Autodesk Fusion 360 part; units mm, degrees
note: some values were not read from the file. Chosen so that the rebuilt part matches the saved one: which bodies a step acts on.
(part 4 of 4)
  line L205 (7.7875, 59.3875) -> (20.7875, 59.3875)
  arc A172 (21.2875, 58.8875) -> (20.7875, 59.3875) centre (20.7875, 58.8875) ccw
  line L206 (21.2875, 58.8875) -> (21.2875, 45.8875)
  arc A173 (20.7875, 45.3875) -> (21.2875, 45.8875) centre (20.7875, 45.8875) ccw
  line L207 (20.7875, 45.3875) -> (7.7875, 45.3875)
  arc A174 (93.0125, 64.9375) -> (93.5125, 64.4375) centre (93.5125, 64.9375) ccw
  line L208 (93.0125, 64.9375) -> (93.0125, 77.9375)
  arc A175 (93.5125, 78.4375) -> (93.0125, 77.9375) centre (93.5125, 77.9375) ccw
  line L209 (93.5125, 78.4375) -> (106.5125, 78.4375)
  arc A176 (107.0125, 77.9375) -> (106.5125, 78.4375) centre (106.5125, 77.9375) ccw
  line L210 (107.0125, 77.9375) -> (107.0125, 64.9375)
  arc A177 (106.5125, 64.4375) -> (107.0125, 64.9375) centre (106.5125, 64.9375) ccw
  line L211 (106.5125, 64.4375) -> (93.5125, 64.4375)
  arc A178 (35.8625, 64.9375) -> (36.3625, 64.4375) centre (36.3625, 64.9375) ccw
  line L212 (35.8625, 64.9375) -> (35.8625, 77.9375)
  arc A179 (36.3625, 78.4375) -> (35.8625, 77.9375) centre (36.3625, 77.9375) ccw
  line L213 (36.3625, 78.4375) -> (49.3625, 78.4375)
  arc A180 (49.8625, 77.9375) -> (49.3625, 78.4375) centre (49.3625, 77.9375) ccw
  line L214 (49.8625, 77.9375) -> (49.8625, 64.9375)
  arc A181 (49.3625, 64.4375) -> (49.8625, 64.9375) centre (49.3625, 64.9375) ccw
  line L215 (49.3625, 64.4375) -> (36.3625, 64.4375)
  arc A182 (131.1125, 64.9375) -> (131.6125, 64.4375) centre (131.6125, 64.9375) ccw
  line L216 (131.1125, 64.9375) -> (131.1125, 77.9375)
  arc A183 (131.6125, 78.4375) -> (131.1125, 77.9375) centre (131.6125, 77.9375) ccw
  line L217 (131.6125, 78.4375) -> (144.6125, 78.4375)
  arc A184 (145.1125, 77.9375) -> (144.6125, 78.4375) centre (144.6125, 77.9375) ccw
  line L218 (145.1125, 77.9375) -> (145.1125, 64.9375)
  arc A185 (144.6125, 64.4375) -> (145.1125, 64.9375) centre (144.6125, 64.9375) ccw
  line L219 (144.6125, 64.4375) -> (131.6125, 64.4375)
  arc A186 (28.7187, 103.0375) -> (29.2188, 102.5375) centre (29.2188, 103.0375) ccw
  line L220 (28.7187, 103.0375) -> (28.7188, 116.0375)
  arc A187 (29.2188, 116.5375) -> (28.7188, 116.0375) centre (29.2188, 116.0375) ccw
  line L221 (29.2188, 116.5375) -> (42.2188, 116.5375)
  arc A188 (42.7188, 116.0375) -> (42.2188, 116.5375) centre (42.2188, 116.0375) ccw
  line L222 (42.7188, 116.0375) -> (42.7188, 103.0375)
  arc A189 (42.2188, 102.5375) -> (42.7188, 103.0375) centre (42.2188, 103.0375) ccw
  line L223 (42.2188, 102.5375) -> (29.2188, 102.5375)
  arc A190 (31.1, 45.8875) -> (31.6, 45.3875) centre (31.6, 45.8875) ccw
  line L224 (31.1, 45.8875) -> (31.1, 58.8875)
  arc A191 (31.6, 59.3875) -> (31.1, 58.8875) centre (31.6, 58.8875) ccw
  line L225 (31.6, 59.3875) -> (44.6, 59.3875)
  arc A192 (45.1, 58.8875) -> (44.6, 59.3875) centre (44.6, 58.8875) ccw
  line L226 (45.1, 58.8875) -> (45.1, 45.8875)
  arc A193 (44.6, 45.3875) -> (45.1, 45.8875) centre (44.6, 45.8875) ccw
  line L227 (44.6, 45.3875) -> (31.6, 45.3875)
  arc A194 (59.675, 26.8375) -> (60.175, 26.3375) centre (60.175, 26.8375) ccw
  line L228 (59.675, 26.8375) -> (59.675, 39.8375)
  arc A195 (60.175, 40.3375) -> (59.675, 39.8375) centre (60.175, 39.8375) ccw
  line L229 (60.175, 40.3375) -> (73.175, 40.3375)
  arc A196 (73.675, 39.8375) -> (73.175, 40.3375) centre (73.175, 39.8375) ccw
  line L230 (73.675, 39.8375) -> (73.675, 26.8375)
  arc A197 (73.175, 26.3375) -> (73.675, 26.8375) centre (73.175, 26.8375) ccw
  line L231 (73.175, 26.3375) -> (60.175, 26.3375)
  arc A198 (2.525, 26.8375) -> (3.025, 26.3375) centre (3.025, 26.8375) ccw
  line L232 (2.525, 26.8375) -> (2.525, 39.8375)
  arc A199 (3.025, 40.3375) -> (2.525, 39.8375) centre (3.025, 39.8375) ccw
  line L233 (3.025, 40.3375) -> (16.025, 40.3375)
  arc A200 (16.525, 39.8375) -> (16.025, 40.3375) centre (16.025, 39.8375) ccw
  line L234 (16.525, 39.8375) -> (16.525, 26.8375)
  arc A201 (16.025, 26.3375) -> (16.525, 26.8375) centre (16.025, 26.8375) ccw
  line L235 (16.025, 26.3375) -> (3.025, 26.3375)
  line L236 (2.3022, 101.2599) -> (40.5603, 101.2599)
  line L237 (40.5603, 101.2599) -> (40.5603, 80.4875)
  line L238 (40.5603, 80.4875) -> (2.3022, 80.4875)
  line L239 (2.3022, 80.4875) -> (2.3022, 101.2599)
  line L240 (79.4039, 119.5375) -> (192.9223, 119.5375)
  line L241 (192.9223, 119.5375) -> (192.9223, 99.5375)
  line L242 (192.9223, 99.5375) -> (79.4039, 99.5375)
  line L243 (79.4039, 99.5375) -> (79.4039, 119.5375)
  line L244 (189.9223, 107.7515) -> (189.9223, 110.0455)
  line L245 (245.1898, 82.2099) -> (283.4478, 82.2099)
  line L246 (283.4478, 82.2099) -> (283.4478, 61.4375)
  line L247 (283.4478, 61.4375) -> (245.1898, 61.4375)
  line L248 (245.1898, 61.4375) -> (245.1898, 82.2099)
  line L249 (248.1898, 71.9455) -> (248.1898, 69.6515)
  line L250 (253.4048, 79.2099) -> (251.3568, 79.2099)
  line L251 (280.4478, 69.6515) -> (280.4478, 71.9455)
  line L252 (257.8188, 64.4375) -> (270.8188, 64.4375)
  line L253 (247.571, 42.896) -> (285.829, 42.896)
  line L254 (285.829, 42.896) -> (285.829, 23.3375)
  line L255 (285.829, 23.3375) -> (247.571, 23.3375)
  line L256 (247.571, 23.3375) -> (247.571, 42.896)
  line L257 (250.571, 33.8455) -> (250.571, 31.5515)
  line L258 (282.829, 31.5515) -> (282.829, 33.8455)
  line L259 (279.662, 41.1099) -> (277.614, 41.1099)
  line L260 (260.2, 26.3375) -> (273.2, 26.3375)
  dimension "d40" = 3
  dimension "d41" = 3
  dimension "d43" = 3
  dimension "d44" = 3
  dimension "d45" = 3
  dimension "d46" = 3
  dimension "d47" = 3
  dimension "d48" = 3
  dimension "d50" = 3
  dimension "d51" = 3
  dimension "d52" = 3
  dimension "d53" = 3
  dimension "d54" = 3
  dimension "d55" = 3
  dimension "d56" = 1.7861
  dimension "d57" = 3
  constraint horizontal L236
  constraint vertical L237
  constraint horizontal L238
  constraint vertical L239
  constraint horizontal L240
  constraint vertical L241
  constraint horizontal L242
  constraint vertical L243
  constraint horizontal L245
  constraint vertical L246
  constraint horizontal L247
  constraint vertical L248
  constraint horizontal L253
  constraint vertical L254
  constraint horizontal L255
  constraint vertical L256
  measures "d40" distance of L108 L238
  measures "d41" distance of L115 L239
  measures "d43" distance of L120 L236
  measures "d44" distance of L101 L237
  measures "d45" distance of L3 L242
  measures "d46" distance of L12 L243
  measures "d47" distance of L21 L240
  measures "d48" distance of L241 L244
  measures "d50" distance of L248 L249
  measures "d51" distance of L245 L250
  measures "d52" distance of L246 L251
  measures "d53" distance of L247 L252
  measures "d54" distance of L256 L257
  measures "d55" distance of L254 L258
  measures "d56" distance of L253 L259
  measures "d57" distance of L255 L260
extrude "Extrude2" cut sketch "Sketch3" against normal blind 1.5 contours L0 L1 L2 A0 L3 A1 L4 L5 A2 L6 A3 L7 A4 L8 L9 A5 L10 L11 A6 L12 A7 L13 A8 L14 A9 L15 A10 L16 A11 L17 A12 L18 A13 L19 L20 A14 L21 A15 L22 L23 L24 L240 L242 L243 | L0 L1 L2 A0 L3 A1 L4 L5 A2 L6 A3 L7 A4 L8 L9 A5 L10 L11 A6 L12 A7 L13 A8 L14 A9 L15 A10 L16 A11 L17 A12 L18 A13 L19 L20 A14 L21 A15 L22 L23 L24 L240 L241 L242 | L236 L237 L238 L239 | L245 L246 L247 L248 | L253 L254 L255 L256 bodies 1 2
sketch "Sketch4" plane through (0, 0, 0) normal (0, 0, -1) x (1, 0, 0)
  arc A0 (2.525, 26.8375) -> (3.025, 26.3375) centre (3.025, 26.8375) ccw
  line L0 (2.525, 26.8375) -> (2.525, 39.8375)
  arc A1 (3.025, 40.3375) -> (2.525, 39.8375) centre (3.025, 39.8375) ccw
  line L1 (3.025, 40.3375) -> (16.025, 40.3375)
  arc A2 (16.525, 39.8375) -> (16.025, 40.3375) centre (16.025, 39.8375) ccw
  line L2 (16.525, 39.8375) -> (16.525, 26.8375)
  arc A3 (16.025, 26.3375) -> (16.525, 26.8375) centre (16.025, 26.8375) ccw
  line L3 (16.025, 26.3375) -> (3.025, 26.3375)
  arc A4 (59.675, 26.8375) -> (60.175, 26.3375) centre (60.175, 26.8375) ccw
  line L4 (59.675, 26.8375) -> (59.675, 39.8375)
  arc A5 (60.175, 40.3375) -> (59.675, 39.8375) centre (60.175, 39.8375) ccw
  line L5 (60.175, 40.3375) -> (73.175, 40.3375)
  arc A6 (73.675, 39.8375) -> (73.175, 40.3375) centre (73.175, 39.8375) ccw
  line L6 (73.675, 39.8375) -> (73.675, 26.8375)
  arc A7 (73.175, 26.3375) -> (73.675, 26.8375) centre (73.175, 26.8375) ccw
  line L7 (73.175, 26.3375) -> (60.175, 26.3375)
  arc A8 (31.1, 45.8875) -> (31.6, 45.3875) centre (31.6, 45.8875) ccw
  line L8 (31.1, 45.8875) -> (31.1, 58.8875)
  arc A9 (31.6, 59.3875) -> (31.1, 58.8875) centre (31.6, 58.8875) ccw
  line L9 (31.6, 59.3875) -> (44.6, 59.3875)
  arc A10 (45.1, 58.8875) -> (44.6, 59.3875) centre (44.6, 58.8875) ccw
  line L10 (45.1, 58.8875) -> (45.1, 45.8875)
  arc A11 (44.6, 45.3875) -> (45.1, 45.8875) centre (44.6, 45.8875) ccw
  line L11 (44.6, 45.3875) -> (31.6, 45.3875)
  arc A12 (28.7187, 103.0375) -> (29.2188, 102.5375) centre (29.2188, 103.0375) ccw
  line L12 (28.7187, 103.0375) -> (28.7188, 116.0375)
  arc A13 (29.2188, 116.5375) -> (28.7188, 116.0375) centre (29.2188, 116.0375) ccw
  line L13 (29.2188, 116.5375) -> (42.2188, 116.5375)
  arc A14 (42.7188, 116.0375) -> (42.2188, 116.5375) centre (42.2188, 116.0375) ccw
  line L14 (42.7188, 116.0375) -> (42.7188, 103.0375)
  arc A15 (42.2188, 102.5375) -> (42.7188, 103.0375) centre (42.2188, 103.0375) ccw
  line L15 (42.2188, 102.5375) -> (29.2188, 102.5375)
  arc A16 (131.1125, 64.9375) -> (131.6125, 64.4375) centre (131.6125, 64.9375) ccw
  line L16 (131.1125, 64.9375) -> (131.1125, 77.9375)
  arc A17 (131.6125, 78.4375) -> (131.1125, 77.9375) centre (131.6125, 77.9375) ccw
  line L17 (131.6125, 78.4375) -> (144.6125, 78.4375)
  arc A18 (145.1125, 77.9375) -> (144.6125, 78.4375) centre (144.6125, 77.9375) ccw
  line L18 (145.1125, 77.9375) -> (145.1125, 64.9375)
  arc A19 (144.6125, 64.4375) -> (145.1125, 64.9375) centre (144.6125, 64.9375) ccw
  line L19 (144.6125, 64.4375) -> (131.6125, 64.4375)
  arc A20 (35.8625, 64.9375) -> (36.3625, 64.4375) centre (36.3625, 64.9375) ccw
  line L20 (35.8625, 64.9375) -> (35.8625, 77.9375)
  arc A21 (36.3625, 78.4375) -> (35.8625, 77.9375) centre (36.3625, 77.9375) ccw
  line L21 (36.3625, 78.4375) -> (49.3625, 78.4375)
  arc A22 (49.8625, 77.9375) -> (49.3625, 78.4375) centre (49.3625, 77.9375) ccw
  line L22 (49.8625, 77.9375) -> (49.8625, 64.9375)
  arc A23 (49.3625, 64.4375) -> (49.8625, 64.9375) centre (49.3625, 64.9375) ccw
  line L23 (49.3625, 64.4375) -> (36.3625, 64.4375)
  arc A24 (93.0125, 64.9375) -> (93.5125, 64.4375) centre (93.5125, 64.9375) ccw
  line L24 (93.0125, 64.9375) -> (93.0125, 77.9375)
  arc A25 (93.5125, 78.4375) -> (93.0125, 77.9375) centre (93.5125, 77.9375) ccw
  line L25 (93.5125, 78.4375) -> (106.5125, 78.4375)
  arc A26 (107.0125, 77.9375) -> (106.5125, 78.4375) centre (106.5125, 77.9375) ccw
  line L26 (107.0125, 77.9375) -> (107.0125, 64.9375)
  arc A27 (106.5125, 64.4375) -> (107.0125, 64.9375) centre (106.5125, 64.9375) ccw
  line L27 (106.5125, 64.4375) -> (93.5125, 64.4375)
  arc A28 (7.2875, 45.8875) -> (7.7875, 45.3875) centre (7.7875, 45.8875) ccw
  line L28 (7.2875, 45.8875) -> (7.2875, 58.8875)
  arc A29 (7.7875, 59.3875) -> (7.2875, 58.8875) centre (7.7875, 58.8875) ccw
  line L29 (7.7875, 59.3875) -> (20.7875, 59.3875)
  arc A30 (21.2875, 58.8875) -> (20.7875, 59.3875) centre (20.7875, 58.8875) ccw
  line L30 (21.2875, 58.8875) -> (21.2875, 45.8875)
  arc A31 (20.7875, 45.3875) -> (21.2875, 45.8875) centre (20.7875, 45.8875) ccw
  line L31 (20.7875, 45.3875) -> (7.7875, 45.3875)
  arc A32 (135.875, 26.8375) -> (136.375, 26.3375) centre (136.375, 26.8375) ccw
  line L32 (135.875, 26.8375) -> (135.875, 39.8375)
  arc A33 (136.375, 40.3375) -> (135.875, 39.8375) centre (136.375, 39.8375) ccw
  line L33 (136.375, 40.3375) -> (149.375, 40.3375)
  arc A34 (149.875, 39.8375) -> (149.375, 40.3375) centre (149.375, 39.8375) ccw
  line L34 (149.875, 39.8375) -> (149.875, 26.8375)
  arc A35 (149.375, 26.3375) -> (149.875, 26.8375) centre (149.375, 26.8375) ccw
  line L35 (149.375, 26.3375) -> (136.375, 26.3375)
  arc A36 (35.8625, 3.025) -> (36.3625, 2.525) centre (36.3625, 3.025) ccw
  line L36 (35.8625, 3.025) -> (35.8625, 16.025)
  arc A37 (36.3625, 16.525) -> (35.8625, 16.025) centre (36.3625, 16.025) ccw
  line L37 (36.3625, 16.525) -> (49.3625, 16.525)
  arc A38 (49.8625, 16.025) -> (49.3625, 16.525) centre (49.3625, 16.025) ccw
  line L38 (49.8625, 16.025) -> (49.8625, 3.025)
  arc A39 (49.3625, 2.525) -> (49.8625, 3.025) centre (49.3625, 3.025) ccw
  line L39 (49.3625, 2.525) -> (36.3625, 2.525)
  arc A40 (73.9625, 64.9375) -> (74.4625, 64.4375) centre (74.4625, 64.9375) ccw
  line L40 (73.9625, 64.9375) -> (73.9625, 77.9375)
  arc A41 (74.4625, 78.4375) -> (73.9625, 77.9375) centre (74.4625, 77.9375) ccw
  line L41 (74.4625, 78.4375) -> (87.4625, 78.4375)
  arc A42 (87.9625, 77.9375) -> (87.4625, 78.4375) centre (87.4625, 77.9375) ccw
  line L42 (87.9625, 77.9375) -> (87.9625, 64.9375)
  arc A43 (87.4625, 64.4375) -> (87.9625, 64.9375) centre (87.4625, 64.9375) ccw
  line L43 (87.4625, 64.4375) -> (74.4625, 64.4375)
  arc A44 (54.9125, 64.9375) -> (55.4125, 64.4375) centre (55.4125, 64.9375) ccw
  line L44 (54.9125, 64.9375) -> (54.9125, 77.9375)
  arc A45 (55.4125, 78.4375) -> (54.9125, 77.9375) centre (55.4125, 77.9375) ccw
  line L45 (55.4125, 78.4375) -> (68.4125, 78.4375)
  arc A46 (68.9125, 77.9375) -> (68.4125, 78.4375) centre (68.4125, 77.9375) ccw
  line L46 (68.9125, 77.9375) -> (68.9125, 64.9375)
  arc A47 (68.4125, 64.4375) -> (68.9125, 64.9375) centre (68.4125, 64.9375) ccw
  line L47 (68.4125, 64.4375) -> (55.4125, 64.4375)
  arc A48 (126.35, 45.8875) -> (126.85, 45.3875) centre (126.85, 45.8875) ccw
  line L48 (126.35, 45.8875) -> (126.35, 58.8875)
  arc A49 (126.85, 59.3875) -> (126.35, 58.8875) centre (126.85, 58.8875) ccw
  line L49 (126.85, 59.3875) -> (139.85, 59.3875)
  arc A50 (140.35, 58.8875) -> (139.85, 59.3875) centre (139.85, 58.8875) ccw
  line L50 (140.35, 58.8875) -> (140.35, 45.8875)
  arc A51 (139.85, 45.3875) -> (140.35, 45.8875) centre (139.85, 45.8875) ccw
  line L51 (139.85, 45.3875) -> (126.85, 45.3875)
  arc A52 (116.825, 26.8375) -> (117.325, 26.3375) centre (117.325, 26.8375) ccw
  line L52 (116.825, 26.8375) -> (116.825, 39.8375)
  arc A53 (117.325, 40.3375) -> (116.825, 39.8375) centre (117.325, 39.8375) ccw
  line L53 (117.325, 40.3375) -> (130.325, 40.3375)
  arc A54 (130.825, 39.8375) -> (130.325, 40.3375) centre (130.325, 39.8375) ccw
  line L54 (130.825, 39.8375) -> (130.825, 26.8375)
  arc A55 (130.325, 26.3375) -> (130.825, 26.8375) centre (130.325, 26.8375) ccw
  line L55 (130.325, 26.3375) -> (117.325, 26.3375)
  arc A56 (107.3, 45.8875) -> (107.8, 45.3875) centre (107.8, 45.8875) ccw
  line L56 (107.3, 45.8875) -> (107.3, 58.8875)
  arc A57 (107.8, 59.3875) -> (107.3, 58.8875) centre (107.8, 58.8875) ccw
  line L57 (107.8, 59.3875) -> (120.8, 59.3875)
  arc A58 (121.3, 58.8875) -> (120.8, 59.3875) centre (120.8, 58.8875) ccw
  line L58 (121.3, 58.8875) -> (121.3, 45.8875)
  arc A59 (120.8, 45.3875) -> (121.3, 45.8875) centre (120.8, 45.8875) ccw
  line L59 (120.8, 45.3875) -> (107.8, 45.3875)
  arc A60 (54.9125, 3.025) -> (55.4125, 2.525) centre (55.4125, 3.025) ccw
  line L60 (54.9125, 3.025) -> (54.9125, 16.025)
  arc A61 (55.4125, 16.525) -> (54.9125, 16.025) centre (55.4125, 16.025) ccw
  line L61 (55.4125, 16.525) -> (68.4125, 16.525)
  arc A62 (68.9125, 16.025) -> (68.4125, 16.525) centre (68.4125, 16.025) ccw
  line L62 (68.9125, 16.025) -> (68.9125, 3.025)
  arc A63 (68.4125, 2.525) -> (68.9125, 3.025) centre (68.4125, 3.025) ccw
  line L63 (68.4125, 2.525) -> (55.4125, 2.525)
  arc A64 (145.4, 45.8875) -> (145.9, 45.3875) centre (145.9, 45.8875) ccw
  line L64 (145.4, 45.8875) -> (145.4, 58.8875)
  arc A65 (145.9, 59.3875) -> (145.4, 58.8875) centre (145.9, 58.8875) ccw
  line L65 (145.9, 59.3875) -> (158.9, 59.3875)
  arc A66 (159.4, 58.8875) -> (158.9, 59.3875) centre (158.9, 58.8875) ccw
  line L66 (159.4, 58.8875) -> (159.4, 45.8875)
  arc A67 (158.9, 45.3875) -> (159.4, 45.8875) centre (158.9, 45.8875) ccw
  line L67 (158.9, 45.3875) -> (145.9, 45.3875)
  arc A68 (93.0125, 3.025) -> (93.5125, 2.525) centre (93.5125, 3.025) ccw
  line L68 (93.0125, 3.025) -> (93.0125, 16.025)
  arc A69 (93.5125, 16.525) -> (93.0125, 16.025) centre (93.5125, 16.025) ccw
  line L69 (93.5125, 16.525) -> (106.5125, 16.525)
  arc A70 (107.0125, 16.025) -> (106.5125, 16.525) centre (106.5125, 16.025) ccw
  line L70 (107.0125, 16.025) -> (107.0125, 3.025)
  arc A71 (106.5125, 2.525) -> (107.0125, 3.025) centre (106.5125, 3.025) ccw
  line L71 (106.5125, 2.525) -> (93.5125, 2.525)
  arc A72 (73.9625, 3.025) -> (74.4625, 2.525) centre (74.4625, 3.025) ccw
  line L72 (73.9625, 3.025) -> (73.9625, 16.025)
  arc A73 (74.4625, 16.525) -> (73.9625, 16.025) centre (74.4625, 16.025) ccw
  line L73 (74.4625, 16.525) -> (87.4625, 16.525)
  arc A74 (87.9625, 16.025) -> (87.4625, 16.525) centre (87.4625, 16.025) ccw
  line L74 (87.9625, 16.025) -> (87.9625, 3.025)
  arc A75 (87.4625, 2.525) -> (87.9625, 3.025) centre (87.4625, 3.025) ccw
  line L75 (87.4625, 2.525) -> (74.4625, 2.525)
  arc A76 (2.525, 3.025) -> (3.025, 2.525) centre (3.025, 3.025) ccw
  line L76 (2.525, 3.025) -> (2.525, 16.025)
  arc A77 (3.025, 16.525) -> (2.525, 16.025) centre (3.025, 16.025) ccw
  line L77 (3.025, 16.525) -> (16.025, 16.525)
  arc A78 (16.525, 16.025) -> (16.025, 16.525) centre (16.025, 16.025) ccw
  line L78 (16.525, 16.025) -> (16.525, 3.025)
  arc A79 (16.025, 2.525) -> (16.525, 3.025) centre (16.025, 3.025) ccw
  line L79 (16.025, 2.525) -> (3.025, 2.525)
  arc A80 (140.6375, 3.025) -> (141.1375, 2.525) centre (141.1375, 3.025) ccw
  line L80 (140.6375, 3.025) -> (140.6375, 16.025)
  arc A81 (141.1375, 16.525) -> (140.6375, 16.025) centre (141.1375, 16.025) ccw
  line L81 (141.1375, 16.525) -> (154.1375, 16.525)
  arc A82 (154.6375, 16.025) -> (154.1375, 16.525) centre (154.1375, 16.025) ccw
  line L82 (154.6375, 16.025) -> (154.6375, 3.025)
  arc A83 (154.1375, 2.525) -> (154.6375, 3.025) centre (154.1375, 3.025) ccw
  line L83 (154.1375, 2.525) -> (141.1375, 2.525)
  arc A84 (78.725, 26.8375) -> (79.225, 26.3375) centre (79.225, 26.8375) ccw
  line L84 (78.725, 26.8375) -> (78.725, 39.8375)
  arc A85 (79.225, 40.3375) -> (78.725, 39.8375) centre (79.225, 39.8375) ccw
  line L85 (79.225, 40.3375) -> (92.225, 40.3375)
  arc A86 (92.725, 39.8375) -> (92.225, 40.3375) centre (92.225, 39.8375) ccw
  line L86 (92.725, 39.8375) -> (92.725, 26.8375)
  arc A87 (92.225, 26.3375) -> (92.725, 26.8375) centre (92.225, 26.8375) ccw
  line L87 (92.225, 26.3375) -> (79.225, 26.3375)
  arc A88 (54.9125, 103.0375) -> (55.4125, 102.5375) centre (55.4125, 103.0375) ccw
  line L88 (54.9125, 103.0375) -> (54.9125, 116.0375)
  arc A89 (55.4125, 116.5375) -> (54.9125, 116.0375) centre (55.4125, 116.0375) ccw
  line L89 (55.4125, 116.5375) -> (68.4125, 116.5375)
  arc A90 (68.9125, 116.0375) -> (68.4125, 116.5375) centre (68.4125, 116.0375) ccw
  line L90 (68.9125, 116.0375) -> (68.9125, 103.0375)
  arc A91 (68.4125, 102.5375) -> (68.9125, 103.0375) centre (68.4125, 103.0375) ccw
  line L91 (68.4125, 102.5375) -> (55.4125, 102.5375)
  arc A92 (21.575, 26.8375) -> (22.075, 26.3375) centre (22.075, 26.8375) ccw
  line L92 (21.575, 26.8375) -> (21.575, 39.8375)
  arc A93 (22.075, 40.3375) -> (21.575, 39.8375) centre (22.075, 39.8375) ccw
  line L93 (22.075, 40.3375) -> (35.075, 40.3375)
  arc A94 (35.575, 39.8375) -> (35.075, 40.3375) centre (35.075, 39.8375) ccw
  line L94 (35.575, 39.8375) -> (35.575, 26.8375)
  arc A95 (35.075, 26.3375) -> (35.575, 26.8375) centre (35.075, 26.8375) ccw
  line L95 (35.075, 26.3375) -> (22.075, 26.3375)
  arc A96 (88.25, 45.8875) -> (88.75, 45.3875) centre (88.75, 45.8875) ccw
  line L96 (88.25, 45.8875) -> (88.25, 58.8875)
  arc A97 (88.75, 59.3875) -> (88.25, 58.8875) centre (88.75, 58.8875) ccw
  line L97 (88.75, 59.3875) -> (101.75, 59.3875)
  arc A98 (102.25, 58.8875) -> (101.75, 59.3875) centre (101.75, 58.8875) ccw
  line L98 (102.25, 58.8875) -> (102.25, 45.8875)
  arc A99 (101.75, 45.3875) -> (102.25, 45.8875) centre (101.75, 45.8875) ccw
  line L99 (101.75, 45.3875) -> (88.75, 45.3875)
  arc A100 (45.3875, 83.9875) -> (45.8875, 83.4875) centre (45.8875, 83.9875) ccw
  line L100 (45.3875, 83.9875) -> (45.3875, 96.9875)
  arc A101 (45.8875, 97.4875) -> (45.3875, 96.9875) centre (45.8875, 96.9875) ccw
  line L101 (45.8875, 97.4875) -> (58.8875, 97.4875)
  arc A102 (59.3875, 96.9875) -> (58.8875, 97.4875) centre (58.8875, 96.9875) ccw
  line L102 (59.3875, 96.9875) -> (59.3875, 83.9875)
  arc A103 (58.8875, 83.4875) -> (59.3875, 83.9875) centre (58.8875, 83.9875) ccw
  line L103 (58.8875, 83.4875) -> (45.8875, 83.4875)
  arc A104 (83.4875, 83.9875) -> (83.9875, 83.4875) centre (83.9875, 83.9875) ccw
  line L104 (83.4875, 83.9875) -> (83.4875, 96.9875)
  arc A105 (83.9875, 97.4875) -> (83.4875, 96.9875) centre (83.9875, 96.9875) ccw
  line L105 (83.9875, 97.4875) -> (96.9875, 97.4875)
  arc A106 (97.4875, 96.9875) -> (96.9875, 97.4875) centre (96.9875, 96.9875) ccw
  line L106 (97.4875, 96.9875) -> (97.4875, 83.9875)
  arc A107 (96.9875, 83.4875) -> (97.4875, 83.9875) centre (96.9875, 83.9875) ccw
  line L107 (96.9875, 83.4875) -> (83.9875, 83.4875)
  arc A108 (64.4375, 83.9875) -> (64.9375, 83.4875) centre (64.9375, 83.9875) ccw
  line L108 (64.4375, 83.9875) -> (64.4375, 96.9875)
  arc A109 (64.9375, 97.4875) -> (64.4375, 96.9875) centre (64.9375, 96.9875) ccw
  line L109 (64.9375, 97.4875) -> (77.9375, 97.4875)
  arc A110 (78.4375, 96.9875) -> (77.9375, 97.4875) centre (77.9375, 96.9875) ccw
  line L110 (78.4375, 96.9875) -> (78.4375, 83.9875)
  arc A111 (77.9375, 83.4875) -> (78.4375, 83.9875) centre (77.9375, 83.9875) ccw
  line L111 (77.9375, 83.4875) -> (64.9375, 83.4875)
  arc A112 (4.9062, 103.0375) -> (5.4062, 102.5375) centre (5.4062, 103.0375) ccw
  line L112 (4.9062, 103.0375) -> (4.9062, 116.0375)
  arc A113 (5.4062, 116.5375) -> (4.9062, 116.0375) centre (5.4062, 116.0375) ccw
  line L113 (5.4062, 116.5375) -> (18.4063, 116.5375)
  arc A114 (18.9063, 116.0375) -> (18.4062, 116.5375) centre (18.4062, 116.0375) ccw
  line L114 (18.9063, 116.0375) -> (18.9062, 103.0375)
  arc A115 (18.4062, 102.5375) -> (18.9063, 103.0375) centre (18.4062, 103.0375) ccw
  line L115 (18.4062, 102.5375) -> (5.4062, 102.5375)
  arc A116 (121.5875, 3.025) -> (122.0875, 2.525) centre (122.0875, 3.025) ccw
  line L116 (121.5875, 3.025) -> (121.5875, 16.025)
  arc A117 (122.0875, 16.525) -> (121.5875, 16.025) centre (122.0875, 16.025) ccw
  line L117 (122.0875, 16.525) -> (135.0875, 16.525)
  arc A118 (135.5875, 16.025) -> (135.0875, 16.525) centre (135.0875, 16.025) ccw
  line L118 (135.5875, 16.025) -> (135.5875, 3.025)
  arc A119 (135.0875, 2.525) -> (135.5875, 3.025) centre (135.0875, 3.025) ccw
  line L119 (135.0875, 2.525) -> (122.0875, 2.525)
  arc A120 (40.625, 26.8375) -> (41.125, 26.3375) centre (41.125, 26.8375) ccw
  line L120 (40.625, 26.8375) -> (40.625, 39.8375)
  arc A121 (41.125, 40.3375) -> (40.625, 39.8375) centre (41.125, 39.8375) ccw
  line L121 (41.125, 40.3375) -> (54.125, 40.3375)
  arc A122 (54.625, 39.8375) -> (54.125, 40.3375) centre (54.125, 39.8375) ccw
  line L122 (54.625, 39.8375) -> (54.625, 26.8375)
  arc A123 (54.125, 26.3375) -> (54.625, 26.8375) centre (54.125, 26.8375) ccw
  line L123 (54.125, 26.3375) -> (41.125, 26.3375)
  arc A124 (112.0625, 64.9375) -> (112.5625, 64.4375) centre (112.5625, 64.9375) ccw
  line L124 (112.0625, 64.9375) -> (112.0625, 77.9375)
  arc A125 (112.5625, 78.4375) -> (112.0625, 77.9375) centre (112.5625, 77.9375) ccw
  line L125 (112.5625, 78.4375) -> (125.5625, 78.4375)
  arc A126 (126.0625, 77.9375) -> (125.5625, 78.4375) centre (125.5625, 77.9375) ccw
  line L126 (126.0625, 77.9375) -> (126.0625, 64.9375)
  arc A127 (125.5625, 64.4375) -> (126.0625, 64.9375) centre (125.5625, 64.9375) ccw
  line L127 (125.5625, 64.4375) -> (112.5625, 64.4375)
  arc A128 (121.5875, 83.9875) -> (122.0875, 83.4875) centre (122.0875, 83.9875) ccw
  line L128 (121.5875, 83.9875) -> (121.5875, 96.9875)
  arc A129 (122.0875, 97.4875) -> (121.5875, 96.9875) centre (122.0875, 96.9875) ccw
  line L129 (122.0875, 97.4875) -> (135.0875, 97.4875)
  arc A130 (135.5875, 96.9875) -> (135.0875, 97.4875) centre (135.0875, 96.9875) ccw
  line L130 (135.5875, 96.9875) -> (135.5875, 83.9875)
  arc A131 (135.0875, 83.4875) -> (135.5875, 83.9875) centre (135.0875, 83.9875) ccw
  line L131 (135.0875, 83.4875) -> (122.0875, 83.4875)
  arc A132 (102.5375, 83.9875) -> (103.0375, 83.4875) centre (103.0375, 83.9875) ccw
  line L132 (102.5375, 83.9875) -> (102.5375, 96.9875)
  arc A133 (103.0375, 97.4875) -> (102.5375, 96.9875) centre (103.0375, 96.9875) ccw
  line L133 (103.0375, 97.4875) -> (116.0375, 97.4875)
  arc A134 (116.5375, 96.9875) -> (116.0375, 97.4875) centre (116.0375, 96.9875) ccw
  line L134 (116.5375, 96.9875) -> (116.5375, 83.9875)
  arc A135 (116.0375, 83.4875) -> (116.5375, 83.9875) centre (116.0375, 83.9875) ccw
  line L135 (116.0375, 83.4875) -> (103.0375, 83.4875)
  arc A136 (9.6688, 64.9375) -> (10.1687, 64.4375) centre (10.1687, 64.9375) ccw
  line L136 (9.6688, 64.9375) -> (9.6687, 77.9375)
  arc A137 (10.1687, 78.4375) -> (9.6688, 77.9375) centre (10.1687, 77.9375) ccw
  line L137 (10.1687, 78.4375) -> (23.1687, 78.4375)
  arc A138 (23.6687, 77.9375) -> (23.1687, 78.4375) centre (23.1687, 77.9375) ccw
  line L138 (23.6687, 77.9375) -> (23.6687, 64.9375)
  arc A139 (23.1687, 64.4375) -> (23.6687, 64.9375) centre (23.1687, 64.9375) ccw
  line L139 (23.1687, 64.4375) -> (10.1687, 64.4375)
  arc A140 (50.15, 45.8875) -> (50.65, 45.3875) centre (50.65, 45.8875) ccw
  line L140 (50.15, 45.8875) -> (50.15, 58.8875)
  arc A141 (50.65, 59.3875) -> (50.15, 58.8875) centre (50.65, 58.8875) ccw
  line L141 (50.65, 59.3875) -> (63.65, 59.3875)
  arc A142 (64.15, 58.8875) -> (63.65, 59.3875) centre (63.65, 58.8875) ccw
  line L142 (64.15, 58.8875) -> (64.15, 45.8875)
  arc A143 (63.65, 45.3875) -> (64.15, 45.8875) centre (63.65, 45.8875) ccw
  line L143 (63.65, 45.3875) -> (50.65, 45.3875)
  arc A144 (140.6375, 83.9875) -> (141.1375, 83.4875) centre (141.1375, 83.9875) ccw
  line L144 (140.6375, 83.9875) -> (140.6375, 96.9875)
  arc A145 (141.1375, 97.4875) -> (140.6375, 96.9875) centre (141.1375, 96.9875) ccw
  line L145 (141.1375, 97.4875) -> (154.1375, 97.4875)
  arc A146 (154.6375, 96.9875) -> (154.1375, 97.4875) centre (154.1375, 96.9875) ccw
  line L146 (154.6375, 96.9875) -> (154.6375, 83.9875)
  arc A147 (154.1375, 83.4875) -> (154.6375, 83.9875) centre (154.1375, 83.9875) ccw
  line L147 (154.1375, 83.4875) -> (141.1375, 83.4875)
  arc A148 (69.2, 45.8875) -> (69.7, 45.3875) centre (69.7, 45.8875) ccw
  line L148 (69.2, 45.8875) -> (69.2, 58.8875)
  arc A149 (69.7, 59.3875) -> (69.2, 58.8875) centre (69.7, 58.8875) ccw
  line L149 (69.7, 59.3875) -> (82.7, 59.3875)
  arc A150 (83.2, 58.8875) -> (82.7, 59.3875) centre (82.7, 58.8875) ccw
  line L150 (83.2, 58.8875) -> (83.2, 45.8875)
  arc A151 (82.7, 45.3875) -> (83.2, 45.8875) centre (82.7, 45.8875) ccw
  line L151 (82.7, 45.3875) -> (69.7, 45.3875)
  arc A152 (97.775, 26.8375) -> (98.275, 26.3375) centre (98.275, 26.8375) ccw
  line L152 (97.775, 26.8375) -> (97.775, 39.8375)
  arc A153 (98.275, 40.3375) -> (97.775, 39.8375) centre (98.275, 39.8375) ccw
  line L153 (98.275, 40.3375) -> (111.275, 40.3375)
  arc A154 (111.775, 39.8375) -> (111.275, 40.3375) centre (111.275, 39.8375) ccw
  line L154 (111.775, 39.8375) -> (111.775, 26.8375)
  arc A155 (111.275, 26.3375) -> (111.775, 26.8375) centre (111.275, 26.8375) ccw
  line L155 (111.275, 26.3375) -> (98.275, 26.3375)
  line L156 (40.5603, 101.2599) -> (40.5603, 80.4875)
  line L157 (40.5603, 80.4875) -> (2.3022, 80.4875)
  line L158 (2.3022, 80.4875) -> (2.3022, 101.2599)
  line L159 (2.3022, 101.2599) -> (40.5603, 101.2599)
  line L160 (79.4039, 119.5375) -> (157, 119.5375)
  line L161 (157, 119.5375) -> (157, 130.1996)
  line L162 (157, 130.1996) -> (107.4, 130.1996)
  arc A156 (107.4, 130.1996) -> (102.4, 125.1996) centre (107.4, 125.1996) ccw
  line L163 (102.4, 125.1996) -> (102.4, 123.1996)
  line L164 (102.4, 123.1996) -> (31, 123.1996)
  line L165 (31, 123.1996) -> (31, 125.1996)
  arc A157 (31, 125.1996) -> (26, 130.1996) centre (26, 125.1996) ccw
  line L166 (26, 130.1996) -> (1, 130.1996)
  arc A158 (1, 130.1996) -> (-4, 125.1996) centre (1, 125.1996) ccw
  line L167 (-4, 125.1996) -> (-4, -5)
  arc A159 (-4, -5) -> (1, -10) centre (1, -5) ccw
  line L168 (1, -10) -> (26, -10)
  arc A160 (26, -10) -> (31, -5) centre (26, -5) ccw
  line L169 (31, -5) -> (31, -3)
  line L170 (31, -3) -> (102.4, -3)
  line L171 (102.4, -3) -> (102.4, -5)
  arc A161 (102.4, -5) -> (107.4, -10) centre (107.4, -5) ccw
  line L172 (107.4, -10) -> (157, -10)
  line L173 (157, -10) -> (157, 21)
  line L174 (157, 21) -> (152.4, 21)
  line L175 (152.4, 21) -> (152.4, 43)
  line L176 (152.4, 43) -> (162, 43)
  line L177 (162, 43) -> (162, 62)
  line L178 (162, 62) -> (147.5, 62)
  line L179 (147.5, 62) -> (147.5, 81)
  line L180 (147.5, 81) -> (157, 81)
  line L181 (157, 81) -> (157, 99.5375)
  line L182 (157, 99.5375) -> (79.4039, 99.5375)
  line L183 (79.4039, 99.5375) -> (79.4039, 119.5375)
  circle A162 centre (291.8, -7.75) radius 1.4
  line L184 (308.8, -5) -> (308.8, 125.1996)
  line L185 (278.8, -10) -> (303.8, -10)
  line L186 (273.8, -3) -> (273.8, -5)
  circle A163 centre (14.25, -7.75) radius 1.4
  dimension "d60" = 2.8
  dimension "d62" = 2.25
  dimension "d65" = 18
  dimension "d66" = 2.8
  dimension "d67" = 16.75
  dimension "d68" = 2.25
  measures "d60" diameter of A162
  measures "d62" distance of A162.centre L185
  measures "d65" distance of A162.centre L186
  measures "d66" diameter of A163
  measures "d67" distance of L169 A163.centre
  measures "d68" distance of L168 A163.centre
extrude "Extrude3" cut sketch "Sketch4" against normal blind 6 contours A162 | A163 bodies 1 2
equation "d38 = ( 312.8 / 2 ) * 1 mm"
equation "d65 = 20 mm - 2 mm"
